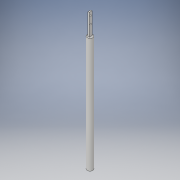
# Autodesk Inventor part: Stereotax adaptor v4
Saved by Autodesk Inventor 2017 (Build 210142000, 142)
## iProperties
Created: 2017-06-29
Part Number: Stereotax adaptor v4
Material: Generic
Document SubType Name: Modeling
Designer: Churlandlab
Density: 1 g/cm^3
Appearance: Default
Author: Churlandlab
Autodesk Inventor part; units mm, degrees
ref_plane "YZ Plane" through (0, 0, 0) normal (1, 0, 0) x (0, 1, 0)
ref_plane "XZ Plane" through (0, 0, 0) normal (0, 1, 0) x (-1, 0, 0)
ref_plane "XY Plane" through (0, 0, 0) normal (0, 0, 1) x (1, 0, 0)
sketch "Sketch1" plane through (0, 0, 0) normal (0, 1, 0) x (-1, 0, 0)
  circle A0 centre (0, 0) radius 3.95
  dimension "d0" = 7.9
  constraints: 1 centre point, 1 coincident
  measures "d0" diameter of A0
extrude "Extrusion1" add sketch "Sketch1" along normal blind 160
sketch "Sketch2" plane through (0, 160, 0) normal (0, 1, 0) x (1, 0, 0)
  line L0 (-0.9, -1.9) -> (0.9, -1.9)
  line L1 (0.9, -1.9) -> (0.9, 1.9)
  line L2 (0.9, 1.9) -> (-0.9, 1.9)
  line L3 (-0.9, 1.9) -> (-0.9, -1.9)
  line L4 (-0.9, -1.9) -> (0.9, 1.9) construction
  line L5 (0.9, -1.9) -> (-0.9, 1.9) construction
  point P0 (0, 0)
  dimension "d3" = 3.8
  dimension "d4" = 1.8
  constraints: 12 end point, 2 midpoint, 2 parallel, 1 horizontal, 1 perpendicular
  measures "d3" distance of L2.end L0.start
  measures "d4" distance of L1.end L2.end
extrude "Extrusion2" add sketch "Sketch2" along normal blind 30
sketch "Sketch3" plane through (0.9, 160, 1.9) normal (1, 0, 0) x (0, 0, -1)
  line L0 (0, 30) -> (3.8, 30) projected
  line L1 (1.9, 30) -> (1.9, 25)
  circle A0 centre (1.9, 25) radius 1.1
  line L2 (1.9, 25) -> (1.9, 15)
  line L3 (3.8, 0) -> (3.8, 30) projected
  circle A1 centre (1.9, 15) radius 1.1
  point P0 (1.9, -160)
  dimension "d7" = 5
  dimension "d8" = 2.2
  dimension "d9" = 10
  dimension "d10" = 2.2
  constraints: 4 end point, 2 centre point, 2 coincident, 1 midpoint, 1 parallel, 1 vertical
  measures "d7" distance of L1.start L1.end
  measures "d8" diameter of A0
  measures "d9" distance of L2.start L2.end
  measures "d10" diameter of A1
hole "Hole1" at (0.9, 185, 0) at (0.9, 175, 0) direction (-1, 0, 0) diameter 2 end through all
body "Solid1"
